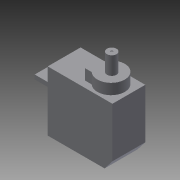
# Autodesk Inventor part: Part1
Saved by Autodesk Inventor 2015 (Build 190159000, 159)
## iProperties
Created: 2015-05-19
Part Number: Part1
Material: Generic
Document SubType Name: Modeling
Designer: Angelina
Density: 1 g/cm^3
Appearance: Default
Author: Angelina
Autodesk Inventor part; units mm, degrees
ref_plane "YZ Plane" through (0, 0, 0) normal (1, 0, 0) x (0, 1, 0)
ref_plane "XZ Plane" through (0, 0, 0) normal (0, 1, 0) x (-1, 0, 0)
ref_plane "XY Plane" through (0, 0, 0) normal (0, 0, 1) x (1, 0, 0)
sketch "Sketch1" plane through (0, 0, 0) normal (0, 0, 1) x (1, 0, 0)
  line L0 (0, 0) -> (23.114, 0)
  line L1 (23.114, 0) -> (23.114, 15.0368)
  line L2 (23.114, 15.0368) -> (0, 15.0368)
  line L3 (0, 15.0368) -> (0, 0)
  dimension "d0" = 15.0368
  dimension "d1" = 23.114
  constraints: 8 end point, 2 parallel, 1 horizontal, 1 perpendicular
  measures "d0" distance of L2.end L0.start
  measures "d1" distance of L0.start L0.end
extrude "Extrusion1" add sketch "Sketch1" along normal blind 11.7348
sketch "Sketch2" plane through (0, 0, 11.7348) normal (0, 0, 1) x (1, 0, 0)
  line L0 (23.114, 0) -> (23.114, 3.6138)
  line L1 (23.114, 0) -> (23.114, 15.0368) projected
  line L2 (0, 0) -> (23.114, 0) projected
  line L3 (20.3034, 0) -> (23.114, 0)
  line L4 (23.114, 3.6138) -> (20.3034, 0)
  constraints: 6 end point, 2 point on line, 1 collinear
extrude "Extrusion2" cut sketch "Sketch2" against normal blind 11.7348
sketch "Sketch3" plane through (0, 0, 11.7348) normal (0, 0, 1) x (1, 0, 0)
  line L0 (-4.6433, 16.5606) -> (27.1067, 16.5606)
  line L1 (27.1067, 16.5606) -> (27.1067, 15.0366)
  line L2 (27.1067, 15.0366) -> (-4.6433, 15.0366)
  line L3 (-4.6433, 15.0366) -> (-4.6433, 16.5606)
  line L4 (23.114, 15.0368) -> (0, 15.0368) projected
  point P0 (0, 0)
  dimension "d6" = 31.75
  dimension "d7" = 1.524
  constraints: 8 end point, 1 horizontal, 1 parallel, 1 perpendicular
  measures "d6" distance of L0.start L0.end
  measures "d7" distance of L0.end L1.end
extrude "Extrusion3" add sketch "Sketch3" against normal blind 11.7348
sketch "Sketch4" plane through (0, 0, 11.7348) normal (0, 0, 1) x (1, 0, 0)
  line L0 (-4.6433, 16.5606) -> (27.1067, 16.5606) projected
  line L1 (0, 16.5606) -> (23.1157, 16.5606)
  line L2 (23.1157, 16.5606) -> (23.1157, 21.3866)
  line L3 (23.1157, 21.3866) -> (0, 21.3866)
  line L4 (0, 21.3866) -> (0, 16.5606)
  point P0 (0, 0)
  dimension "d10" = 4.826
  constraints: 8 end point, 2 parallel, 1 horizontal, 1 perpendicular, 1 point on line
  measures "d10" distance of L1.end L2.end
extrude "Extrusion4" add sketch "Sketch4" against normal up to surface (11.7348 mm away)
sketch "Sketch5" plane through (0, 21.3866, 11.7348) normal (0, 1, 0) x (1, 0, 0)
  circle A0 centre (16.764, 5.8674) radius 4.8959
  line L0 (0, 11.7348) -> (23.1157, 11.7348) projected
  line L1 (0, 0) -> (0, 11.7348) projected
  line L2 (23.1157, 0) -> (0, 0) projected
  line L3 (23.1157, 0) -> (23.1157, 11.7348) projected
  point P0 (0, 11.7348)
  dimension "d14" = 9.7917
  dimension "d39" = 11.7348
  dimension "d40" = 5.8674
  dimension "d46" = 16.764
  constraints: 1 centre point
  measures "d14" diameter of A0
  measures "d39" distance of L2.start L0.end
  measures "d40" distance from line of L0 A0.centre
  measures "d46" distance from line of L1 A0.centre
extrude "Extrusion5" add sketch "Sketch5" along normal blind 3.81 contours A0
sketch "Sketch6" plane through (16.764, 25.1966, 5.8674) normal (0, 1, 0) x (1, 0, 0)
  circle A0 centre (0, 0) radius 4.8958 projected
  arc A1 (-4.5107, 1.9034) -> (-5.2123, 0) centre (-4.8064, 0.9314) ccw
  line L0 (-5.2123, 0) -> (-5.7995, 0)
  line L1 (-5.7995, 0) -> (-5.7995, -3.5655)
  line L2 (-5.7995, -3.5655) -> (-3.355, -3.5655)
  line L3 (-4.228, 0.0962) -> (-4.228, 0.1127)
  point P0 (-16.764, 5.8674)
  point P1 (-5.5059, 0)
  dimension "d35" = 2.4445
  dimension "d36" = 3.5655
  dimension "d37" = 1.016
  dimension "d38" = 0.9314
  constraints: 8 end point, 6 point on circle, 2 parallel, 1 centre point, 1 horizontal, 1 horizontal alignment, 1 midpoint, 1 perpendicular
  measures "d35" distance of L1.end L2.end
  measures "d36" distance of L0.end L1.end
  measures "d37" radius of A1
  measures "d38" distance from line of A1.centre L0
extrude "Extrusion6" add sketch "Sketch6" against normal blind 3.9878 contours A0 L2 L1 L0 A1
sketch "Sketch7" plane through (0, 25.1966, 11.7348) normal (0, 1, 0) x (1, 0, 0)
  circle A0 centre (16.9713, 5.8977) radius 1.7145
  point P0 (0, 11.7348)
  dimension "d19" = 3.429
  constraints: 1 centre point, 1 coincident
  measures "d19" diameter of A0
extrude "Extrusion7" add sketch "Sketch7" along normal blind 6.35
sketch "Sketch8" plane through (16.9713, 31.5466, 5.8371) normal (0, 1, 0) x (1, 0, 0)
  circle A0 centre (0, 0) radius 0.41
  point P0 (-16.9713, 5.8371)
  constraints: 1 centre point
extrude "Extrusion8" cut sketch "Sketch8" against normal blind 0.254
sketch "Sketch9" plane through (-4.6433, 16.5606, 11.7348) normal (0, 1, 0) x (1, 0, 0)
  line L0 (4.6433, 0) -> (4.6433, 11.7348) projected
  line L1 (0, 0) -> (0, 11.7348) projected
  line L2 (31.75, 0) -> (31.75, 11.7348) projected
  line L3 (27.759, 0) -> (27.759, 11.7348) projected
  circle A0 centre (2.3241, 5.8674) radius 1.524
  line L4 (0, 0) -> (4.6433, 0) projected
  circle A1 centre (29.7561, 5.8674) radius 1.524
  line L5 (27.759, 11.7348) -> (31.75, 11.7348) projected
  dimension "d24" = 4.6433
  dimension "d25" = 3.991
  dimension "d26" = 3.048
  dimension "d27" = 2.3241
  dimension "d28" = 11.7348
  dimension "d29" = 5.8674
  dimension "d30" = 3.048
  dimension "d31" = 5.8674
  dimension "d32" = 1.9939
  constraints: 2 centre point
  measures "d24" distance between parallel lines of L0 L1
  measures "d25" distance between parallel lines of L2 L3
  measures "d26" diameter of A0
  measures "d27" distance from line of L1 A0.centre
  measures "d28" distance of L1.start L1.end
  measures "d29" distance from line of L4 A0.centre
  measures "d30" diameter of A1
  measures "d31" distance from line of L5 A1.centre
  measures "d32" distance from line of L2 A1.centre
extrude "Extrusion9" cut sketch "Sketch9" against normal blind 25.4
sketch "Sketch11" plane through (-4.6433, 16.5606, 11.7348) normal (0, 1, 0) x (1, 0, 0)
  circle A0 centre (29.7561, 5.8674) radius 1.524 projected
  circle A1 centre (29.7561, 5.8674) radius 1.524 projected
  line L0 (27.759, 11.7348) -> (27.759, 0) projected
  line L1 (27.759, 0) -> (31.75, 0) projected
  line L2 (31.75, 0) -> (31.75, 11.7348) projected
  line L3 (27.759, 11.7348) -> (31.75, 11.7348) projected
  point P0 (4.6433, 11.7348)
extrude "Extrusion10" cut sketch "Sketch11" against normal blind 25.4
body "Solid1"
